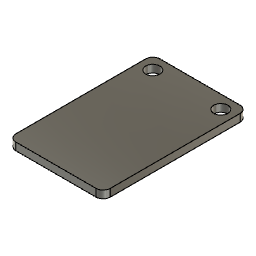
USB-Module CH340G v2 (Autodesk Fusion 360 design; units mm, degrees)
Autodesk Fusion 360 part; units mm, degrees
sketch "Sketch1" plane through (0, 0, 0) normal (0, 0, 1) x (1, 0, 0)
  line L0 (0, 0) -> (20, 0)
  line L1 (20, 0) -> (20, 30.5)
  line L2 (20, 30.5) -> (0, 30.5)
  line L3 (0, 30.5) -> (0, 0)
  line L4 (10, 30.5) -> (10, 0) construction
  circle A0 centre (2.8, 27.7) radius 1.5
  circle A1 centre (17.2, 27.7) radius 1.5
  dimension "d1" = 20
  dimension "d2" = 30.5
  dimension "d5" = 3
  dimension "d6" = 7.2
  dimension "d7" = 2.8
  constraint horizontal L0
  constraint vertical L1
  constraint horizontal L2
  constraint vertical L3
  constraint coincident L0.start L3.end
  constraint midpoint L2 L4.start
  constraint midpoint L0 L4.end
  constraint symmetric L4 A0 A1
  measures "d1" distance of L0.start L0.end
  measures "d2" distance of L0.start L2.end
  measures "d5" diameter of A0
  measures "d6" distance of L4 A0.centre
  measures "d7" distance of L2 A0.centre
extrude "Extrude1" add sketch "Sketch1" along normal blind 1.6
fillet "Fillet1" radius 1.5 4 edges at (0, 30.5, 0.8) (20, 30.5, 0.8) (0, 0, 0.8) (20, 0, 0.8)
equation "d6 = ( 14.4 / 2 ) * 1 mm"
